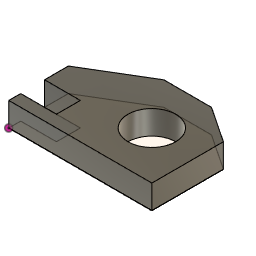
ch2Excercises v7 (Autodesk Fusion 360 design; units mm, degrees)
Autodesk Fusion 360 part; units mm, degrees
sketch "Sketch1" plane through (0, 0, 0) normal (0, 0, 1) x (1, 0, 0) in component "ch2-1"
  line L0 (31.75, 50.8) -> (57.15, 50.8)
  line L1 (57.15, 50.8) -> (76.2, 38.1)
  line L2 (76.2, 38.1) -> (76.2, 0)
  line L3 (76.2, 0) -> (0, 0)
  line L4 (0, 0) -> (0, 6.35)
  line L5 (0, 6.35) -> (19.05, 6.35)
  line L6 (19.05, 6.35) -> (19.05, 19.05)
  line L7 (19.05, 19.05) -> (0, 19.05)
  line L8 (0, 19.05) -> (0, 31.75)
  line L9 (0, 31.75) -> (31.75, 50.8)
  dimension "d1" = 25.4
  dimension "d2" = 19.05
  dimension "d3" = 38.1
  dimension "d4" = 12.7
  dimension "d5" = 19.05
  dimension "d6" = 76.2
  dimension "d7" = 6.35
  dimension "d8" = 50.8
  dimension "d9" = 31.75
  constraint horizontal L0
  constraint vertical L2
  constraint perpendicular L3 L4
  constraint perpendicular L2 L5
  constraint perpendicular L5 L6
  constraint perpendicular L6 L7
  constraint perpendicular L2 L3
  constraint equal L5 L7
  constraint perpendicular L7 L8
  constraint coincident L3.end L4.start
  measures "d1" distance of L0.start L0.end
  measures "d2" horizontal distance of L0.end L1.end
  measures "d3" distance of L1.end L2.end
  measures "d4" distance of L5.end L6.end
  measures "d5" distance of L4.end L5.end
  measures "d6" distance of L2.end L3.end
  measures "d7" distance of L3.end L4.end
  measures "d8" vertical distance of L0.end L2.end
  measures "d9" distance of L3.end L8.end
extrude "Extrude1" add sketch "Sketch1" along normal blind 12.7 makes body 1 in component "ch2-1"
sketch "Sketch2" plane through (0, 0, 12.7) normal (0, 0, 1) x (-1, 0, 0) in component "ch2-1"
  line L0 (0, -31.75) -> (0, -19.05)
  line L1 (0, -19.05) -> (-19.05, -19.05)
  line L2 (-19.05, -19.05) -> (-19.05, -6.35)
  line L3 (-19.05, -6.35) -> (0, -6.35)
  line L4 (0, -6.35) -> (0, 0)
  line L5 (0, 0) -> (-76.2, 0)
  line L6 (-76.2, 0) -> (-76.2, -38.1)
  line L7 (-76.2, -38.1) -> (-57.15, -50.8)
  line L8 (-57.15, -50.8) -> (-31.75, -50.8)
  line L9 (-31.75, -50.8) -> (0, -31.75)
  circle A0 centre (-50.8, -25.4) radius 12.7
  dimension "d12" = 25.4
  dimension "d13" = 25.4
  dimension "d14" = 25.4
  measures "d12" diameter of A0
  measures "d13" distance of L6 A0.centre
  measures "d14" distance of L5 A0.centre
extrude "Extrude2" cut sketch "Sketch2" against normal through all contours A0 bodies 1 in component "ch2-1"
sketch "Sketch1 (2)" plane through (0, 0, 0) normal (0, 0, 1) x (1, 0, 0) in component "ch2-2"
  line L0 (0, 165.1) -> (0, 0)
  line L1 (0, 0) -> (139.7, 0)
  line L2 (139.7, 0) -> (139.7, 63.5)
  line L3 (139.7, 63.5) -> (203.2, 63.5)
  line L4 (203.2, 63.5) -> (203.2, 139.7)
  line L5 (203.2, 139.7) -> (165.1, 165.1)
  line L6 (165.1, 165.1) -> (0, 165.1)
  dimension "d16" = 165.1
  dimension "d17" = 203.2
  dimension "d18" = 63.5
  dimension "d19" = 63.5
  dimension "d20" = 165.1
  dimension "d21" = 139.7
  constraint vertical L0
  constraint perpendicular L0 L1
  constraint perpendicular L1 L2
  constraint perpendicular L2 L3
  constraint perpendicular L1 L4
  constraint perpendicular L0 L6
  constraint coincident L0.end L1.start
  measures "d16" distance of L0.start L5.end
  measures "d17" horizontal distance of L0.end L3.end
  measures "d18" distance of L2.end L3.end
  measures "d19" distance of L1.end L2.end
  measures "d20" distance of L0.start L0.end
  measures "d21" vertical distance of L1.end L4.end
extrude "Extrude1'" add sketch "Sketch1 (2)" along normal blind 3.175 separate body makes body 2 in component "ch2-2"
sketch "Sketch2 (2)" plane through (0, 0, 3.175) normal (0, 0, 1) x (-1, 0, 0) in component "ch2-2"
  line L0 (-165.1, -165.1) -> (0, -165.1)
  line L1 (0, -165.1) -> (0, 0)
  line L2 (0, 0) -> (-139.7, 0)
  line L3 (-139.7, 0) -> (-139.7, -63.5)
  line L4 (-139.7, -63.5) -> (-203.2, -63.5)
  line L5 (-203.2, -63.5) -> (-203.2, -139.7)
  line L6 (-203.2, -139.7) -> (-165.1, -165.1)
  circle A0 centre (-127, -127) radius 19.05
  circle A1 centre (-63.5, -76.2) radius 31.75
  dimension "d24" = 38.1
  dimension "d25" = 63.5
  dimension "d26" = 127
  dimension "d27" = 38.1
  dimension "d28" = 63.5
  dimension "d29" = 76.2
  measures "d24" diameter of A0
  measures "d25" diameter of A1
  measures "d26" distance of L1 A0.centre
  measures "d27" distance of L0 A0.centre
  measures "d28" distance of L1 A1.centre
  measures "d29" distance of L2 A1.centre
extrude "Extrude2'" cut sketch "Sketch2 (2)" against normal through all contours A0 | A1 bodies 2 in component "ch2-2"
sketch "Sketch1 (3)" plane through (0, 0, 0) normal (0, 1, 0) x (1, 0, 0) in component "ch2-3"
  line L0 (0, 0) -> (101.6, 0)
  line L1 (101.6, 0) -> (101.6, -44.45)
  line L2 (101.6, -44.45) -> (66.675, -63.5)
  line L3 (66.675, -63.5) -> (34.925, -63.5)
  line L4 (34.925, -63.5) -> (0, -44.45)
  line L5 (0, -44.45) -> (0, 0)
  dimension "d31" = 101.6
  dimension "d32" = 31.75
  dimension "d33" = 44.45
  dimension "d34" = 63.5
  constraint horizontal L0
  constraint perpendicular L0 L1
  constraint perpendicular L1 L3
  constraint perpendicular L0 L5
  constraint equal L2 L4
  constraint equal L1 L5
  constraint coincident L0.start L5.end
  measures "d31" distance of L0.start L0.end
  measures "d32" distance of L2.end L3.end
  measures "d33" distance of L0.end L1.end
  measures "d34" vertical distance of L0.start L3.end
extrude "Extrude1''" add sketch "Sketch1 (3)" along normal blind 6.35 separate body makes body 3 in component "ch2-3"
sketch "Sketch2 (3)" plane through (0, 0, 0) normal (0, -1, 0) x (1, 0, 0) in component "ch2-3"
  line L0 (34.925, 63.5) -> (0, 44.45)
  line L1 (0, 44.45) -> (0, 0)
  line L2 (0, 0) -> (101.6, 0)
  line L3 (101.6, 0) -> (101.6, 44.45)
  line L4 (101.6, 44.45) -> (66.675, 63.5)
  line L5 (66.675, 63.5) -> (34.925, 63.5)
  circle A0 centre (50.8, 31.75) radius 15.875
  circle A1 centre (82.55, 19.05) radius 6.35
  circle A2 centre (19.05, 19.05) radius 6.35
  dimension "d37" = 31.75
  dimension "d38" = 12.7
  dimension "d39" = 12.7
  dimension "d40" = 19.05
  dimension "d41" = 19.05
  dimension "d42" = 19.05
  dimension "d43" = 19.05
  dimension "d44" = 31.75
  dimension "d45" = 50.8
  measures "d37" diameter of A0
  measures "d38" diameter of A1
  measures "d39" diameter of A2
  measures "d40" distance of L1 A2.centre
  measures "d41" distance of L2 A2.centre
  measures "d42" distance of L3 A1.centre
  measures "d43" distance of L2 A1.centre
  measures "d44" distance of L2 A0.centre
  measures "d45" distance of L1 A0.centre
extrude "Extrude2''" cut sketch "Sketch2 (3)" against normal through all contours A0 | A1 | A2 bodies 3 in component "ch2-3"
sketch "Sketch1 (4)" plane through (0, 0, 0) normal (0, 0, 1) x (1, 0, 0) in component "ch2-6"
  circle A0 centre (0, 0) radius 88.9
  dimension "d47" = 177.8
  constraint coincident A0.centre origin
  measures "d47" diameter of A0
extrude "Extrude1'''" add sketch "Sketch1 (4)" along normal blind 6.35 separate body makes body 4 in component "ch2-6"
sketch "Sketch2 (4)" plane through (0, 0, 6.35) normal (0, 0, 1) x (-1, 0, 0) in component "ch2-6"
  circle A0 centre (0, 0) radius 88.9
  circle A1 centre (0, 0) radius 34.925
  dimension "d50" = 69.85
  constraint concentric A0 A1
  measures "d50" diameter of A1
extrude "Extrude2'''" add sketch "Sketch2 (4)" along normal blind 6.35 contours A1 bodies 4 in component "ch2-6"
sketch "Sketch3" plane through (0, 0, 12.7) normal (0, 0, 1) x (-1, 0, 0) in component "ch2-6"
  circle A0 centre (0, 0) radius 34.925
  circle A1 centre (0, 0) radius 25.4
  dimension "d53" = 50.8
  constraint concentric A0 A1
  measures "d53" diameter of A1
extrude "Extrude3" cut sketch "Sketch3" against normal through all contours A1 bodies 4 in component "ch2-6"
sketch "Sketch4" plane through (0, 0, 6.35) normal (0, 0, 1) x (-1, 0, 0) in component "ch2-6"
  circle A0 centre (0, 0) radius 34.925
  circle A1 centre (0, 0) radius 88.9
  circle A2 centre (0, 0) radius 63.5 construction
  line L0 (0, 0) -> (0, -63.5) construction
  line L1 (0, 0) -> (0, 63.5) construction
  circle A3 centre (0, 63.5) radius 12.7
  dimension "d55" = 127
  dimension "d56" = 25.4
  constraint concentric A0 A2
  constraint coincident A0.centre A1.centre
  constraint coincident A2 L0.end
  constraint vertical L0
  constraint coincident A2 L1.end
  constraint parallel L0 L1
  constraint coincident L1.end A3.centre
  measures "d55" diameter of A2
  measures "d56" diameter of A3
extrude "Extrude4" cut sketch "Sketch4" against normal through all contours A3 bodies 4 in component "ch2-6"
pattern_circular "C-Pattern1" count 3 over 360 about axis through (0, 0, 6.35) along (0, 0, 1) of "Extrude4" in component "ch2-6"
sketch "Sketch1 (5)" plane through (0, 0, 0) normal (0, 1, 0) x (1, 0, 0) in component "ch2-5"
  line L0 (0, 0) -> (114.3, 0)
  line L1 (114.3, 0) -> (114.3, -25.4)
  line L2 (114.3, -25.4) -> (37.3103, -69.85)
  line L3 (37.3103, -69.85) -> (-19.05, -32.9956)
  line L4 (-19.05, -32.9956) -> (0, 0)
  line L5 (114.3, -25.4) -> (114.3, -65.1324) construction
  line L6 (0, 0) -> (-37.4762, 0) construction
  dimension "d60" = 88.9
  dimension "d61" = 114.3
  dimension "d62" = 60
  dimension "d63" = 60
  dimension "d64" = 38.1
  dimension "d65" = 25.4
  constraint horizontal L0
  constraint perpendicular L0 L1
  constraint parallel L1 L5
  constraint parallel L0 L6
  constraint coincident L0.start L4.end
  measures "d60" distance of L1.end L2.end
  measures "d61" distance of L0.start L0.end
  measures "d62" angle of L2 L5
  measures "d63" angle of L4 L6
  measures "d64" distance of L0.start L3.end
  measures "d65" distance of L0.end L1.end
extrude "Extrude1''''" add sketch "Sketch1 (5)" along normal blind 6.35 separate body makes body 5 in component "ch2-5"
sketch "Sketch2 (5)" plane through (0, 0, 0) normal (0, -1, 0) x (1, 0, 0) in component "ch2-5"
  line L0 (37.3103, 69.85) -> (-19.05, 32.9956)
  line L1 (-19.05, 32.9956) -> (0, 0)
  line L2 (0, 0) -> (114.3, 0)
  line L3 (114.3, 0) -> (114.3, 25.4)
  line L4 (114.3, 25.4) -> (37.3103, 69.85)
  circle A0 centre (25.4, 25.4) radius 12.7
  circle A1 centre (88.9, 12.7) radius 6.35
  dimension "d68" = 25.4
  dimension "d69" = 12.7
  dimension "d70" = 88.9
  dimension "d71" = 25.4
  dimension "d72" = 25.4
  dimension "d73" = 12.7
  measures "d68" diameter of A0
  measures "d69" diameter of A1
  measures "d70" horizontal distance of L2.end A0.centre
  measures "d71" distance of L2 A0.centre
  measures "d72" horizontal distance of L2.end A1.centre
  measures "d73" distance of L2 A1.centre
extrude "Extrude2''''" cut sketch "Sketch2 (5)" against normal through all contours A0 | A1 bodies 5 in component "ch2-5"
sketch "Sketch1 (6)" plane through (0, 0, 0) normal (0, 1, 0) x (1, 0, 0) in component "ch2-4"
  line L0 (0, 0) -> (95.25, 0)
  line L1 (95.25, 0) -> (81.1867, -24.3583)
  line L2 (81.1867, -24.3583) -> (38.1, -44.45)
  line L3 (38.1, -44.45) -> (19.05, -44.45)
  line L4 (19.05, -44.45) -> (19.05, -31.75)
  line L5 (19.05, -31.75) -> (0, -31.75)
  line L6 (0, -31.75) -> (0, 0)
  line L7 (38.1, -44.45) -> (81.28, -44.45) construction
  dimension "d75" = 95.25
  dimension "d76" = 60
  dimension "d77" = 25
  dimension "d78" = 38.1
  dimension "d79" = 19.05
  dimension "d80" = 31.75
  dimension "d81" = 44.45
  constraint coincident L0.start L6.end
  constraint horizontal L0
  constraint parallel L0 L3
  constraint perpendicular L3 L4
  constraint perpendicular L4 L5
  constraint perpendicular L0 L6
  constraint parallel L3 L7
  measures "d75" distance of L0.start L0.end
  measures "d76" angle of L0 L1
  measures "d77" angle of L2 L7
  measures "d78" horizontal distance of L2.end L5.end
  measures "d79" distance of L4.end L5.end
  measures "d80" distance of L0.start L5.end
  measures "d81" vertical distance of L0.start L3.end
extrude "Extrude1'''''" add sketch "Sketch1 (6)" along normal blind 6.35 separate body makes body 6 in component "ch2-4"
sketch "Sketch2 (6)" plane through (0, 6.35, 0) normal (0, 1, 0) x (-1, 0, 0) in component "ch2-4"
  line L0 (0, 31.75) -> (-19.05, 31.75)
  line L1 (-19.05, 31.75) -> (-19.05, 44.45)
  line L2 (-19.05, 44.45) -> (-38.1, 44.45)
  line L3 (-38.1, 44.45) -> (-81.1867, 24.3583)
  line L4 (-81.1867, 24.3583) -> (-95.25, 0)
  line L5 (-95.25, 0) -> (0, 0)
  line L6 (0, 0) -> (0, 31.75)
  line L7 (0, 0) -> (-6.35, 0)
  line L8 (-6.35, 0) -> (-6.35, 31.7537)
  line L9 (-6.35, 31.7537) -> (0, 31.75)
  line L10 (0, 31.75) -> (0, 0)
  dimension "d84" = 6.35
  constraint coincident L5.end L6.start
  constraint perpendicular L6 L7
  constraint vertical L8
  constraint coincident L0.start L6.end
  constraint equal L7 L9
  measures "d84" distance of L5.end L7.end
extrude "Extrude2'''''" add sketch "Sketch2 (6)" along normal blind 25.4 contours L0 L5 L6 L7 L8 L10 bodies 6 in component "ch2-4"
sketch "Sketch3 (2)" plane through (0, 31.75, 0) normal (0, 1, 0) x (-1, 0, 0) in component "ch2-4"
  line L0 (0, 31.75) -> (-6.35, 31.75)
  line L1 (-6.35, 31.75) -> (-6.35, 0)
  line L2 (-6.35, 0) -> (0, 0)
  line L3 (0, 0) -> (0, 31.75)
  line L4 (-19.05, 31.75) -> (0, 31.75)
  line L5 (0, 31.75) -> (0, 0)
  line L6 (0, 0) -> (-95.25, 0)
  line L7 (-95.25, 0) -> (-81.1867, 24.3583)
  line L8 (-81.1867, 24.3583) -> (-38.1, 44.45)
  line L9 (-38.1, 44.45) -> (-19.05, 44.45)
  line L10 (-19.05, 44.45) -> (-19.05, 31.75)
extrude "Extrude3'" add sketch "Sketch3 (2)" along normal blind 6.35 bodies 6 in component "ch2-4"
sketch "Sketch4 (2)" plane through (6.35, 0, 0) normal (1, 0, 0) x (0, 1, 0) in component "ch2-4"
  line L0 (6.35, 31.75) -> (6.35, 0)
  line L1 (6.35, 0) -> (31.75, 0)
  line L2 (31.75, 0) -> (31.75, 31.75)
  line L3 (31.75, 31.75) -> (6.35, 31.75)
  line L4 (6.35, 0) -> (6.35, 6.35)
  line L5 (6.35, 6.35) -> (31.75, 6.35)
  line L6 (31.75, 6.35) -> (31.75, 0)
  line L7 (31.75, 0) -> (6.35, 0)
  dimension "d89" = 6.35
  dimension "d90" = 25.4
  constraint coincident L0.end L1.start
  constraint perpendicular L1 L4
  constraint perpendicular L4 L5
  constraint coincident L1.end L2.start
  measures "d89" distance of L0.end L4.end
  measures "d90" distance of L4.end L5.end
extrude "Extrude4'" add sketch "Sketch4 (2)" along normal blind 88.9 contours L0 L1 L2 L4 L5 L6 L7 bodies 6 in component "ch2-4"
extrude "Extrude5" cut 1 faces at (94.0279, 6.35, 4.2333) along direction (0, 1, 0) up to surface (25.4 mm away) on bodies 6 bodies 6 in component "ch2-4"
sketch "Sketch5" plane through (0, 0, 0) normal (0, -1, 0) x (1, 0, 0) in component "ch2-4"
  line L0 (19.05, 31.75) -> (0, 31.75)
  line L1 (0, 31.75) -> (0, 0)
  line L2 (0, 0) -> (95.25, 0)
  line L3 (95.25, 0) -> (81.1867, 24.3583)
  line L4 (81.1867, 24.3583) -> (38.1, 44.45)
  line L5 (38.1, 44.45) -> (19.05, 44.45)
  line L6 (19.05, 44.45) -> (19.05, 31.75)
  circle A0 centre (38.1, 19.05) radius 9.525
  dimension "d95" = 19.05
  dimension "d96" = 19.05
  dimension "d97" = 38.1
  measures "d95" diameter of A0
  measures "d96" distance of L2 A0.centre
  measures "d97" distance of L1 A0.centre
extrude "Extrude6" cut sketch "Sketch5" against normal through all contours A0 bodies 6 in component "ch2-4"
component "ch2-1" placed x (1, 0, 0) y (0, 1, 0) z (0, 0, 1) at (0, 0, 0)
component "ch2-2" placed x (1, 0, 0) y (0, 1, 0) z (0, 0, 1) at (0, 0, 0)
component "ch2-3" placed x (1, 0, 0) y (0, 1, 0) z (0, 0, 1) at (0, 0, 0)
component "ch2-4" placed x (1, 0, 0) y (0, 1, 0) z (0, 0, 1) at (0, 0, 0)
component "ch2-5" placed x (1, 0, 0) y (0, 1, 0) z (0, 0, 1) at (0, 0, 0)
component "ch2-6" placed x (1, 0, 0) y (0, 1, 0) z (0, 0, 1) at (0, 0, 0)
